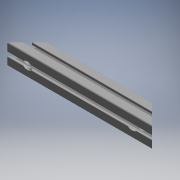
# Autodesk Inventor part: GFBL85050-250-SET_b
Saved by Autodesk Inventor 2017.3 (Build 213256000, 256)
## iProperties
Part Number: GFBL85050-250-SET_b
Material: Generic
Catalog Web Link: www.cadenas.de
Description: GFBL8-4545,GFBL8-4590,GFBL8-5050,GFBL8-50100_body-Brackets for Reinforcement - HFS8-45 Series-
Vendor: MISUMI
Document SubType Name: Modeling
Designer: partserver
Manufacturer: MISUMI
Mass: 488.007 g
Surface Area: 1242.44 cm^2
Volume: 488.007 cm^3
Density: 1 g/cm^3
Appearance: PSOLRGB-192-192-192
Category: PARTsolutions
Company: MISUMI
Title: GFBL85050-250-SET
Author: Cadenas PARTsolutions
Comments: Brackets for Reinforcement - HFS8-45 Series-
PSOL_IDENT_0: {$CADENAS_DATA\23d-libs\misumi\metric\38_al_extrusions_blackets\8_45\gfbl8_45\gfbl8_45_body.prj},226
PSOL_IDENT_1: {VTYP=3D},{NB=GFBL85050-250-SET_b},{LINA=GFBL85050-250-SET},{NN=GFBL8-4545,GFBL8-4590,GFBL8-5050,GF
PSOL_IDENT_2: BL8-50100_body},{DATE=08.06.2021 08:26:11},{GEOMDATE=23.05.2017 06:09:00},{VERSION=},{LINEID=30},{WB
PSOL_IDENT_3: VAR=L,ALT1},{WBNUMERIC=L}  {NB=GFBL85050-250-SET_b},{LINA=GFBL85050-250-SET},{KT=DUMMY},{PN=GFBL8505
PSOL_IDENT_4: 0-250-SET},{TYPE=GFBL8},{NO=5050},{L=250},{ALT1=-SET}
NB: GFBL85050-250-SET_b
NN: GFBL8-4545,GFBL8-4590,GFBL8-5050,GFBL8-50100_body
NT: Brackets for Reinforcement - HFS8-45 Series-
NBSYN: $PN._b
LINA: GFBL85050-250-SET
CATALOG: Misumi
PN: GFBL85050-250-SET
TYPE: GFBL8
NO: 5050
L: 250
ALT1: SET Applicable Screws and Nuts Set
SUPPLIER: MISUMI
ARTICLENO: GFBL85050-250-SET_b
BOMINFO: GFBL85050-250-SET
CREATOR: CADENAS GmbH
Autodesk Inventor part; units mm, degrees
sketch "_____3" plane through (0, 0, 0) normal (1, 0, 0) x (0, 0, -1)
  arc A0 (-25, -22) -> (-22, -25) centre (-22, -22) ccw
  line L0 (-22, -25) -> (-6, -25)
  arc A1 (-6, -25) -> (-5, -24) centre (-6, -24) ccw
  line L1 (-5, -24) -> (-5, -20)
  arc A2 (-5, -20) -> (-6, -19) centre (-6, -20) ccw
  line L2 (-6, -19) -> (-10, -19)
  line L3 (-10, -19) -> (-10, -14.62)
  line L4 (-10, -14.62) -> (-7.38, -12)
  line L5 (-7.38, -12) -> (-1.3464, -12)
  arc A3 (-1.3464, -12) -> (-1.0964, -11.933) centre (-1.3464, -11.5) ccw
  line L6 (-1.0964, -11.933) -> (0, -11.3)
  line L7 (0, -11.3) -> (0.9624, -11.8557)
  arc A4 (0.9624, -11.8557) -> (1.4624, -11.8557) centre (1.2124, -11.4226) ccw
  line L8 (1.4624, -11.8557) -> (1.7049, -11.7157)
  line L9 (1.7049, -11.7157) -> (3.5, -12)
  line L10 (3.5, -12) -> (7.38, -12)
  line L11 (7.38, -12) -> (10, -14.62)
  line L12 (10, -14.62) -> (10, -19)
  line L13 (10, -19) -> (6, -19)
  arc A5 (6, -19) -> (5, -20) centre (6, -20) ccw
  line L14 (5, -20) -> (5, -24)
  arc A6 (5, -24) -> (6, -25) centre (6, -24) ccw
  line L15 (6, -25) -> (22, -25)
  arc A7 (22, -25) -> (25, -22) centre (22, -22) ccw
  line L16 (25, -22) -> (25, -6)
  arc A8 (25, -6) -> (24, -5) centre (24, -6) ccw
  line L17 (24, -5) -> (20, -5)
  arc A9 (20, -5) -> (19, -6) centre (20, -6) ccw
  line L18 (19, -6) -> (19, -10)
  line L19 (19, -10) -> (14.62, -10)
  line L20 (14.62, -10) -> (12, -7.38)
  line L21 (12, -7.38) -> (12, -1.3464)
  arc A10 (12, -1.3464) -> (11.933, -1.0964) centre (11.5, -1.3464) ccw
  line L22 (11.933, -1.0964) -> (11.3, 0)
  line L23 (11.3, 0) -> (11.8557, 0.9624)
  arc A11 (11.8557, 0.9624) -> (11.8557, 1.4624) centre (11.4226, 1.2124) ccw
  line L24 (11.8557, 1.4624) -> (11.7157, 1.7049)
  line L25 (11.7157, 1.7049) -> (12, 3.5)
  line L26 (12, 3.5) -> (12, 7.38)
  line L27 (12, 7.38) -> (14.62, 10)
  line L28 (14.62, 10) -> (19, 10)
  line L29 (19, 10) -> (19, 6)
  arc A12 (19, 6) -> (20, 5) centre (20, 6) ccw
  line L30 (20, 5) -> (24, 5)
  arc A13 (24, 5) -> (25, 6) centre (24, 6) ccw
  line L31 (25, 6) -> (25, 22)
  arc A14 (25, 22) -> (22, 25) centre (22, 22) ccw
  line L32 (22, 25) -> (6, 25)
  arc A15 (6, 25) -> (5, 24) centre (6, 24) ccw
  line L33 (5, 24) -> (5, 20)
  arc A16 (5, 20) -> (6, 19) centre (6, 20) ccw
  line L34 (6, 19) -> (10, 19)
  line L35 (10, 19) -> (10, 14.62)
  line L36 (10, 14.62) -> (7.38, 12)
  line L37 (7.38, 12) -> (1.3464, 12)
  arc A17 (1.3464, 12) -> (1.0964, 11.933) centre (1.3464, 11.5) ccw
  line L38 (1.0964, 11.933) -> (0, 11.3)
  line L39 (0, 11.3) -> (-0.9624, 11.8557)
  arc A18 (-0.9624, 11.8557) -> (-1.4624, 11.8557) centre (-1.2124, 11.4226) ccw
  line L40 (-1.4624, 11.8557) -> (-1.7049, 11.7157)
  line L41 (-1.7049, 11.7157) -> (-3.5, 12)
  line L42 (-3.5, 12) -> (-7.38, 12)
  line L43 (-7.38, 12) -> (-10, 14.62)
  line L44 (-10, 14.62) -> (-10, 19)
  line L45 (-10, 19) -> (-6, 19)
  arc A19 (-6, 19) -> (-5, 20) centre (-6, 20) ccw
  line L46 (-5, 20) -> (-5, 24)
  arc A20 (-5, 24) -> (-6, 25) centre (-6, 24) ccw
  line L47 (-6, 25) -> (-22, 25)
  arc A21 (-22, 25) -> (-25, 22) centre (-22, 22) ccw
  line L48 (-25, 22) -> (-25, 6)
  arc A22 (-25, 6) -> (-24, 5) centre (-24, 6) ccw
  line L49 (-24, 5) -> (-20, 5)
  arc A23 (-20, 5) -> (-19, 6) centre (-20, 6) ccw
  line L50 (-19, 6) -> (-19, 10)
  line L51 (-19, 10) -> (-14.62, 10)
  line L52 (-14.62, 10) -> (-12, 7.38)
  line L53 (-12, 7.38) -> (-12, 1.3464)
  arc A24 (-12, 1.3464) -> (-11.933, 1.0964) centre (-11.5, 1.3464) ccw
  line L54 (-11.933, 1.0964) -> (-11.3, 0)
  line L55 (-11.3, 0) -> (-11.8557, -0.9624)
  arc A25 (-11.8557, -0.9624) -> (-11.8557, -1.4624) centre (-11.4226, -1.2124) ccw
  line L56 (-11.8557, -1.4624) -> (-11.7157, -1.7049)
  line L57 (-11.7157, -1.7049) -> (-12, -3.5)
  line L58 (-12, -3.5) -> (-12, -7.38)
  line L59 (-12, -7.38) -> (-14.62, -10)
  line L60 (-14.62, -10) -> (-19, -10)
  line L61 (-19, -10) -> (-19, -6)
  arc A26 (-19, -6) -> (-20, -5) centre (-20, -6) ccw
  line L62 (-20, -5) -> (-24, -5)
  arc A27 (-24, -5) -> (-25, -6) centre (-24, -6) ccw
  line L63 (-25, -6) -> (-25, -22)
  circle A28 centre (0, 0) radius 5.25
  constraints: 128 end point, 56 point on circle, 29 centre point
extrude "Extrusion1" add sketch "_____3" along normal blind 353.5534
sketch "_____6" plane through (0, 0, 0) normal (0, 0, 1) x (1, 0, 0)
  circle A0 centre (176.7767, 151.7767) radius 260
  line L0 (0, -25) -> (353.5534, -25)
  line L1 (353.5534, -25) -> (176.7767, 151.7767)
  line L2 (176.7767, 151.7767) -> (0, -25)
  constraints: 6 end point, 1 centre point
extrude "Extrusion2" cut sketch "_____6" along normal mid plane 150
sketch "_____11" plane through (0, 0, 0) normal (0, 0, 1) x (1, 0, 0)
  line L0 (329.0092, -0.4558) -> (272.4407, -57.0244)
  line L1 (290.8255, -38.6396) -> (284.4615, -32.2756)
  line L2 (284.4615, -32.2756) -> (316.2813, -0.4558)
  line L3 (316.2813, -0.4558) -> (319.4633, -3.6378)
  line L4 (319.4633, -3.6378) -> (325.8273, 2.7261)
  line L5 (325.8273, 2.7261) -> (329.0092, -0.4558)
  line L6 (329.0092, -0.4558) -> (290.8255, -38.6396)
  constraints: 14 end point
revolve "Revolution1" cut sketch "_____11" angle 360 about axis through (329.0092, -0.4558, 0) along (0.7071068, 0.7071068, 0)
sketch "_____12" plane through (0, 0, 0) normal (0, 0, 1) x (1, 0, 0)
  line L0 (81.1127, -57.0244) -> (24.5442, -0.4558)
  line L1 (24.5442, -0.4558) -> (27.7261, 2.7261)
  line L2 (27.7261, 2.7261) -> (34.0901, -3.6378)
  line L3 (34.0901, -3.6378) -> (37.2721, -0.4558)
  line L4 (37.2721, -0.4558) -> (69.0919, -32.2756)
  line L5 (69.0919, -32.2756) -> (62.7279, -38.6396)
  line L6 (62.7279, -38.6396) -> (24.5442, -0.4558)
  constraints: 14 end point
revolve "Revolution2" cut sketch "_____12" angle 360 about axis through (81.1127, -57.0244, 0) along (0.7071068, -0.7071068, 0)
ref_plane "to_bolt21_XY" through (30.9079, -6.82, 0) normal (0.7071068, -0.7071068, 0) x (0, 0, -1)
ref_plane "to_bolt21_YZ" through (30.9079, -6.82, 0) normal (0, 0, -1) x (0.7071068, 0.7071068, 0)
ref_plane "to_bolt21_ZX" through (30.9079, -6.82, 0) normal (0.7071068, 0.7071068, 0) x (0.7071068, -0.7071068, 0)
ref_plane "to_bolt22_XY" through (322.6455, -6.82, 0) normal (-0.7071068, -0.7071068, 0) x (0, 0, -1)
ref_plane "to_bolt22_YZ" through (322.6455, -6.82, 0) normal (0, 0, -1) x (0.7071068, -0.7071068, 0)
ref_plane "to_bolt22_ZX" through (322.6455, -6.82, 0) normal (0.7071068, -0.7071068, 0) x (-0.7071068, -0.7071068, 0)
ref_plane "to_bolt23_XY" through (30.9079, -6.82, 50) normal (0.7071068, -0.7071068, 0) x (0, 0, -1)
ref_plane "to_bolt23_YZ" through (30.9079, -6.82, 50) normal (0, 0, -1) x (0.7071068, 0.7071068, 0)
ref_plane "to_bolt23_ZX" through (30.9079, -6.82, 50) normal (0.7071068, 0.7071068, 0) x (0.7071068, -0.7071068, 0)
ref_plane "to_bolt24_XY" through (322.6455, -6.82, 50) normal (-0.7071068, -0.7071068, 0) x (0, 0, -1)
ref_plane "to_bolt24_YZ" through (322.6455, -6.82, 50) normal (0, 0, -1) x (0.7071068, -0.7071068, 0)
ref_plane "to_bolt24_ZX" through (322.6455, -6.82, 50) normal (0.7071068, -0.7071068, 0) x (-0.7071068, -0.7071068, 0)
ref_plane "to_nut21_XY" through (30.9079, -6.82, 0) normal (0.7071068, -0.7071068, 0) x (0, 0, -1)
ref_plane "to_nut21_YZ" through (30.9079, -6.82, 0) normal (0, 0, -1) x (0.7071068, 0.7071068, 0)
ref_plane "to_nut21_ZX" through (30.9079, -6.82, 0) normal (0.7071068, 0.7071068, 0) x (0.7071068, -0.7071068, 0)
ref_plane "to_nut22_XY" through (322.6455, -6.82, 0) normal (-0.7071068, -0.7071068, 0) x (0, 0, -1)
ref_plane "to_nut22_YZ" through (322.6455, -6.82, 0) normal (0, 0, -1) x (0.7071068, -0.7071068, 0)
ref_plane "to_nut22_ZX" through (322.6455, -6.82, 0) normal (0.7071068, -0.7071068, 0) x (-0.7071068, -0.7071068, 0)
ref_plane "to_nut23_XY" through (30.9079, -6.82, 50) normal (0.7071068, -0.7071068, 0) x (0, 0, -1)
ref_plane "to_nut23_YZ" through (30.9079, -6.82, 50) normal (0, 0, -1) x (0.7071068, 0.7071068, 0)
ref_plane "to_nut23_ZX" through (30.9079, -6.82, 50) normal (0.7071068, 0.7071068, 0) x (0.7071068, -0.7071068, 0)
ref_plane "to_nut24_XY" through (322.6455, -6.82, 50) normal (-0.7071068, -0.7071068, 0) x (0, 0, -1)
ref_plane "to_nut24_YZ" through (322.6455, -6.82, 50) normal (0, 0, -1) x (0.7071068, -0.7071068, 0)
ref_plane "to_nut24_ZX" through (322.6455, -6.82, 50) normal (0.7071068, -0.7071068, 0) x (-0.7071068, -0.7071068, 0)
body "Solid1"
